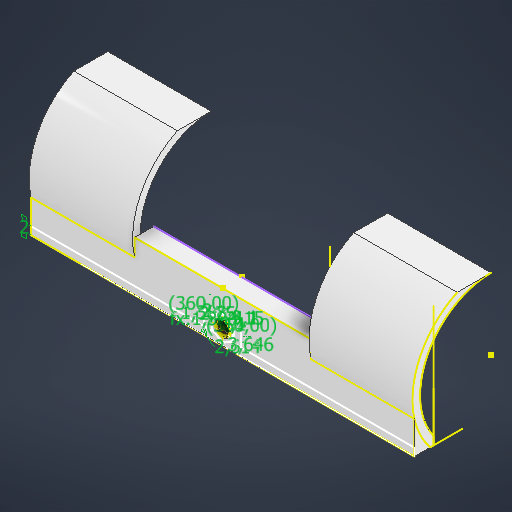
# Autodesk Inventor part: main body wheels part
Saved by Autodesk Inventor 2026.2 (Build 302298010, 298A)
## iProperties
Created: 2026-04-17
Part Number: main body wheels part
Material: Generic
Document SubType Name: Modeling
Designer: Martin
Density: 1 g/cm^3
Appearance: Bronze - Satin
Author: Martin
Autodesk Inventor part; units mm, degrees
ref_plane "YZ Plane" through (0, 0, 0) normal (1, 0, 0) x (0, 1, 0)
ref_plane "XZ Plane" through (0, 0, 0) normal (0, 1, 0) x (-1, 0, 0)
ref_plane "XY Plane" through (0, 0, 0) normal (0, 0, 1) x (1, 0, 0)
sketch "Sketch1" plane through (0, 0, 0) normal (1, 0, 0) x (0, 1, 0)
  circle A0 centre (0, 0) radius 15
  line L0 (-13, -15) -> (-13, 85)
  arc A1 (18.5, 0) -> (-10.8282, 15) centre (0, 0) ccw
  arc A2 (18.5, 8.8318) -> (-13, 15.8509) centre (0, 0) ccw
  line L1 (18.5, 25) -> (18.5, -15) construction
  line L2 (0, 15) -> (-13, 15)
  line L3 (-10.5, 15) -> (-7.5, 15)
  line L4 (-7.5, 15) -> (-7.5, 24)
  line L5 (-7.5, 24) -> (-10.5, 24)
  line L6 (-10.5, 24) -> (-10.5, 15)
  line L7 (18.5, 8.8318) -> (18.5, 0)
  line L8 (-9, 24) -> (-9, 15) construction
  arc A3 (-10.8282, 15) -> (-13, 13.1624) centre (0, 0) ccw
  point P0 (0, -15)
  point P1 (-13, 7.4833)
  dimension "d0" = 30
  dimension "d1" = 2
  dimension "d3" = 100
  dimension "d4" = 37
  dimension "d5" = 41
  dimension "d7" = 3
  dimension "d8" = 9
  dimension "d9" = 2.5
  dimension "d10" = 15
  dimension "d11" = 40
  dimension "d12" = 18.5
  constraints: 18 end point, 9 point on circle, 6 point on line, 4 centre point, 3 coincident, 2 horizontal alignment, 2 midpoint, 2 parallel, 2 perpendicular, 2 tangent, 2 vertical, 1 horizontal
  measures "d0" diameter of A0
  measures "d1" distance edge to line of A0 L0
  measures "d3" distance of L0.start L0.end
  measures "d4" diameter of A1
  measures "d5" diameter of A2
  measures "d7" distance of L5.end L4.end
  measures "d8" distance of L5.end L3.start
  measures "d9" distance between parallel lines of L0 L6
  measures "d10" vertical distance of point (0, 0) L0.start
  measures "d11" distance of L1.end L1.start
  measures "d12" distance of A0.start L1.end
extrude "Extrusion1" add sketch "Sketch1" along normal mid plane 100 contours A0 L0 | A0 L0
extrude "Extrusion2" add sketch "Sketch1" along normal mid plane 49 contours A0 L0 A3 L2 | L0 L2 A3
sketch "Sketch2" plane through (-24.5, -13, 15) normal (0, 0, 1) x (1, 0, 0)
  circle A0 centre (24.5, 4) radius 1.5
  point P0 (24.5, 13)
  constraints: 1 centre point
extrude "Extrusion3" add sketch "Sketch2" along normal blind 9
sketch "Sketch3" plane through (-24.5, -13, 15) normal (0, 0, 1) x (1, 0, 0)
  circle A0 centre (24.5, 4) radius 1.5 projected
  circle A1 centre (24.5, 4) radius 1.55
  circle A2 centre (24.5, 4) radius 2.05
  point P0 (24.5, 13)
  dimension "d25" = 3.1
  dimension "d26" = 4.1
  constraints: 4 coincident, 2 centre point
  measures "d25" diameter of A1
  measures "d26" diameter of A2
extrude "Extrusion4" add sketch "Sketch3" along normal blind 5 separate body contours A2
extrude "Extrusion5" cut sketch "Sketch1" along normal mid plane 50 contours A0 L0 | A0 L0 bodies 1
extrude "Extrusion6" add sketch "Sketch1" against normal blind 27 from surface at 50 separate body contours L4 A2 L7 A1 | A1 L6 A2 L4 | L0 A2 L6 A1 L2
extrude "Extrusion7" add sketch "Sketch1" along normal blind 27 from surface at -50 contours L4 A2 L7 A1 | A1 L6 A2 L4 | L0 A2 L6 A1 L2 bodies 3
sketch "Sketch4" plane through (-24.5, -13, 15) normal (0, 0, 1) x (1, 0, 0)
  circle A0 centre (24.5, 4) radius 2.075
  line L0 (1.5, 2.1718) -> (1.5, 0) projected
  line L1 (47.5, 31.5) -> (47.5, 0) projected
  line L2 (1.5, 0) -> (47.5, 0)
  line L3 (47.5, 0) -> (47.5, 13)
  line L4 (47.5, 13) -> (1.5, 13)
  line L5 (1.5, 13) -> (1.5, 0)
  point P0 (24.5, 13)
  point P1 (47.5, 0)
  dimension "d30" = 4.15
  constraints: 8 end point, 2 parallel, 1 centre point, 1 horizontal, 1 perpendicular, 1 point on line
  measures "d30" diameter of A0
sketch "Sketch5" plane through (50, -13, 15) normal (1, 0, 0) x (0, 0, -1)
  arc A0 (6.1682, 31.5) -> (-0.8509, 0) centre (15, 13) ccw projected
  arc A1 (15, 31.5) -> (0, 2.1718) centre (15, 13) ccw projected
  line L0 (0, 0) -> (-0.8509, 0) projected
  line L1 (0, 0) -> (7.5167, 0) projected
  line L2 (0, 2.1718) -> (0, 0) projected
  line L3 (0, 31.5) -> (0, 0) projected
  line L4 (0, 13) -> (0, 0) projected
extrude "Extrusion8" add sketch "Sketch4" along normal blind 5 bodies 3
sketch "Sketch6" plane through (23, -13, 20) normal (1, 0, 0) x (0, 0, -1)
  arc A0 (11.1682, 31.5) -> (4.1491, 0) centre (20, 13) ccw projected
  line L0 (4.1491, 0) -> (0, 0) projected
  line L1 (0, 0) -> (0, 8.5)
  line L2 (0, 13) -> (0, 8.5) projected
  line L3 (0, 0) -> (4.1491, 0)
  constraints: 4 end point, 1 collinear, 1 perpendicular, 1 point on circle
extrude "Extrusion9" add sketch "Sketch6" along normal blind 27 bodies 3
extrude "Extrusion10" add sketch "Sketch6" against normal blind 27 from surface at -46 bodies 3
sketch "Sketch7" plane through (23, 18.5, 0) normal (-1, 0, 0) x (0, 0, 1)
  arc A0 (18.5, -18.5) -> (0, 0) centre (0, -18.5) ccw projected
  line L0 (8.8318, 0) -> (0, 0) projected
  arc A1 (15.8509, -31.5) -> (8.8318, 0) centre (0, -18.5) ccw projected
  line L1 (0, 0) -> (-21, 0)
  circle A2 centre (0, -18.5) radius 18.5
  constraints: 2 end point, 1 centre point, 1 coincident, 1 concentric, 1 point on line, 1 tangent
sketch "Sketch8" plane through (-24.5, -13, 20) normal (0, 0, 1) x (1, 0, 0)
  line L0 (21.75, 5.5875) -> (21.75, 2.4125)
  line L1 (21.75, 2.4125) -> (21.75, 5.5875)
  circle A0 centre (24.5, 4) radius 2.075 projected
  line L2 (-25.5, 8.5) -> (1.5, 8.5) projected
  line L3 (-25.5, 8.5) -> (-25.5, 0) projected
  line L4 (74.5, 0) -> (-25.5, 0) projected
  line L5 (74.5, 8.5) -> (74.5, 0) projected
  line L6 (47.5, 8.5) -> (74.5, 8.5) projected
  line L7 (47.5, 13) -> (47.5, 8.5) projected
  line L8 (47.5, 13) -> (1.5, 13) projected
  line L9 (1.5, 8.5) -> (1.5, 13) projected
  circle A1 centre (24.5, 4) radius 2.05 projected
  circle A2 centre (24.5, 4) radius 1.55 projected
  circle A3 centre (24.5, 4) radius 1.5 projected
  line L10 (21.7502, 2.4122) -> (24.4998, 0.8247)
  line L11 (24.5002, 0.8247) -> (27.2498, 2.4122)
  line L12 (27.25, 2.4125) -> (27.25, 5.5875)
  line L13 (27.2498, 5.5878) -> (24.5002, 7.1753)
  line L14 (24.4998, 7.1753) -> (21.7502, 5.5878)
  line L15 (74.5, 0) -> (-25.5, 0)
  line L16 (-25.5, 0) -> (-25.5, 2)
  line L17 (74.5, 2) -> (74.5, 0)
  line L18 (27.2498, 5.5878) -> (21.7502, 2.4122) construction
  line L19 (27.2498, 5.5878) -> (27.25, 5.5879)
  line L20 (24.5, 4) -> (27.25, 2.4125) construction
  line L21 (27.25, 2.4125) -> (27.2502, 2.4124)
  line L22 (27.35, 5.6457) -> (27.35, 2.3548)
  line L23 (24.4998, 7.291) -> (27.3498, 5.6456)
  line L24 (21.6498, 5.6453) -> (24.4998, 7.2908)
  line L25 (21.65, 2.3543) -> (21.65, 5.6452)
  line L26 (24.5002, 0.709) -> (21.6502, 2.3544)
  line L27 (27.3502, 2.3547) -> (24.5002, 0.7092)
  line L28 (26.7359, 2) -> (74.5, 2)
  line L29 (-25.5, 2) -> (22.2641, 2)
  line L30 (29.35, 2) -> (29.35, 5.6456)
  line L31 (29.35, 5.6456) -> (27.3498, 5.6456)
  line L32 (19.65, 2) -> (19.65, 5.6452)
  line L33 (19.65, 5.6452) -> (21.65, 5.6452)
  point P0 (24.5, 13)
  dimension "d45" = 360
  dimension "d47" = 1.5875
  dimension "d48" = 1.5875
  dimension "d49" = 2.75
  dimension "d50" = 2
  dimension "d51" = 0.1
  dimension "d54" = 360
  dimension "d56" = 2.0002
  dimension "d57" = 3.6456
  dimension "d58" = 2.6141
  dimension "d59" = 2
  constraints: 52 end point, 7 point on line, 5 perpendicular, 4 parallel, 1 collinear, 1 horizontal, 1 vertical, 38 other
  measures "d47" vertical distance of A1.centre L0.start
  measures "d48" vertical distance of L0.end point (24.5, 4)
  measures "d49" distance from line of A0.centre L0
  measures "d50" distance of L15.end L16.end
  measures "d51" distance between parallel lines of L12 L22
  measures "d56" distance of L30.end L23.end
  measures "d57" distance of L30.start L30.end
  measures "d58" distance of L28.start L30.start
  measures "d59" distance of L32.end L25.end
equation "\"d48\" = d47"
body "Solid3"
